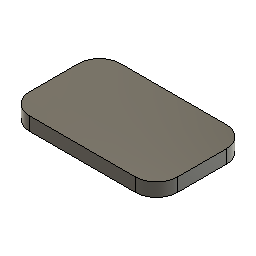
TinyNES_Foam_Cutout_A (Autodesk Fusion 360 design; units mm, degrees)
Autodesk Fusion 360 part; units mm, degrees
sketch "Sketch1" plane through (0, 0, 0) normal (0, 1, 0) x (1, 0, 0)
  line L0 (0, 0) -> (170, 0)
  line L1 (170, 0) -> (170, 170)
  line L2 (170, 170) -> (0, 170)
  line L3 (0, 170) -> (0, 0)
  line L4 (85, 170) -> (85, 128.5) construction
  line L5 (110, 107) -> (60, 107)
  line L6 (50, 117) -> (50, 140)
  line L7 (60, 150) -> (110, 150)
  line L8 (120, 140) -> (120, 117)
  line L9 (120, 107) -> (50, 150) construction
  line L10 (50, 107) -> (120, 150) construction
  arc A0 (60, 150) -> (50, 140) centre (60, 140) ccw
  arc A1 (120, 140) -> (110, 150) centre (110, 140) ccw
  arc A2 (110, 107) -> (120, 117) centre (110, 117) ccw
  arc A3 (50, 117) -> (60, 107) centre (60, 117) ccw
  line L11 (85, 128.5) -> (0, 128.5) construction
  line L12 (85, 128.5) -> (170, 128.5) construction
  arc A4 (0, 108.5) -> (0, 148.5) centre (0, 128.5) ccw
  arc A5 (170, 148.5) -> (170, 108.5) centre (170, 128.5) ccw
  line L13 (85, 0) -> (85, 53.5) construction
  line L14 (140, 20) -> (30, 20)
  line L15 (20, 30) -> (20, 87)
  line L16 (20, 87) -> (150, 87)
  line L17 (150, 87) -> (150, 30)
  line L18 (150, 20) -> (20, 87) construction
  line L19 (20, 20) -> (150, 87) construction
  arc A6 (20, 30) -> (30, 20) centre (30, 30) ccw
  arc A7 (140, 20) -> (150, 30) centre (140, 30) ccw
  line L20 (85, 53.5) -> (20, 53.5) construction
  line L21 (85, 53.5) -> (150, 53.5) construction
  line L22 (20, 53.5) -> (13.5, 53.5) construction
  line L23 (13.5, 53.5) -> (13.5, 64)
  line L24 (13.5, 53.5) -> (13.5, 43)
  line L25 (13.5, 43) -> (13.5, 36.5) construction
  line L26 (13.5, 36.5) -> (20, 36.5) construction
  line L27 (13.5, 64) -> (13.5, 70.5) construction
  line L28 (13.5, 70.5) -> (20, 70.5) construction
  line L29 (13.5, 64) -> (20, 70.5)
  line L30 (13.5, 43) -> (20, 36.5)
  line L31 (156.5, 64) -> (150, 70.5)
  line L32 (156.5, 53.5) -> (156.5, 64)
  line L33 (156.5, 53.5) -> (156.5, 43)
  line L34 (156.5, 43) -> (150, 36.5)
  line L35 (20, 87) -> (20, 85) construction
  line L36 (20, 85) -> (30, 85) construction
  arc A8 (37.0711, 92.0711) -> (20, 85) centre (30, 85) ccw
  line L37 (30, 85) -> (37.0711, 92.0711) construction
  line L38 (30, 85) -> (20, 85) construction
  line L39 (37.0711, 92.0711) -> (42.1421, 87)
  arc A9 (150, 85) -> (132.9289, 92.0711) centre (140, 85) ccw
  line L40 (132.9289, 92.0711) -> (127.8579, 87)
  point P0 (85, 128.5)
  point P1 (85, 53.5)
  dimension "d1" = 170
  dimension "d2" = 170
  dimension "d19" = 41.5
  dimension "d20" = 70
  dimension "d21" = 43
  dimension "d22" = 10
  dimension "d23" = 10
  dimension "d24" = 10
  dimension "d25" = 10
  dimension "d26" = 20
  dimension "d27" = 20
  dimension "d28" = 53.5
  dimension "d29" = 130
  dimension "d30" = 67
  dimension "d31" = 10
  dimension "d32" = 10
  dimension "d33" = 6.5
  dimension "d34" = 10.5
  dimension "d35" = 10.5
  dimension "d36" = 6.5
  dimension "d37" = 6.5
  dimension "d38" = 2
  dimension "d39" = 10
  dimension "d40" = 135
  constraint horizontal L0
  constraint vertical L1
  constraint horizontal L2
  constraint vertical L3
  constraint coincident L0.start L3.end
  constraint midpoint L2 L4.start
  constraint perpendicular L2 L4
  constraint horizontal L5
  constraint perpendicular L5 L6
  constraint parallel L5 L7
  constraint parallel L6 L8
  constraint coincident L9 P0
  constraint coincident L10 P0
  constraint coincident P0 L4.end
  constraint coincident L9.end L6
  constraint coincident L9.end L7
  constraint tangent L6 A0
  constraint tangent L7 A0
  constraint coincident L10.end L7
  constraint coincident L10.end L8
  constraint tangent L7 A1
  constraint tangent L8 A1
  constraint coincident L9.start L8
  constraint coincident L9.start L5
  constraint tangent L8 A2
  constraint tangent L5 A2
  constraint coincident L10.start L6
  constraint coincident L10.start L5
  constraint tangent L6 A3
  constraint tangent L5 A3
  constraint coincident L3 L11.end
  constraint perpendicular L3 L11
  constraint coincident L1 L12.end
  constraint perpendicular L1 L12
  constraint coincident L11.end A4.centre
  constraint coincident L12.end A5.centre
  constraint midpoint L0 L13.start
  constraint perpendicular L0 L13
  constraint horizontal L14
  constraint perpendicular L14 L15
  constraint parallel L14 L16
  constraint parallel L15 L17
  constraint coincident L18 P1
  constraint coincident L19 P1
  constraint coincident P1 L13.end
  constraint coincident L19.start L15
  constraint coincident L19.start L14
  constraint tangent L15 A6
  constraint tangent L14 A6
  constraint coincident L18.start L14
  constraint coincident L18.start L17
  constraint tangent L14 A7
  constraint tangent L17 A7
  constraint coincident L15 L20.end
  constraint perpendicular L15 L20
  constraint coincident L17 L21.end
  constraint perpendicular L17 L21
  constraint perpendicular L15 L22
  constraint perpendicular L22 L23
  constraint perpendicular L22 L24
  constraint parallel L24 L25
  constraint coincident L15 L26.end
  constraint perpendicular L15 L26
  constraint perpendicular L22 L27
  constraint coincident L15 L28.end
  constraint perpendicular L15 L28
  constraint symmetric L13 L22.end L32.start
  constraint symmetric L13 L23.end L31.start
  constraint symmetric L13 L24.end L33.end
  constraint symmetric L13 L26.end L34.end
  constraint symmetric L13 L28.end L31.end
  constraint perpendicular L16 L35
  constraint perpendicular L15 L36
  constraint coincident L36.end A8.centre
  constraint coincident L16 L39.end
  constraint tangent A8 L39
  constraint symmetric L13 L35.end A9.start
  constraint symmetric L13 A8.start A9.end
  constraint symmetric L13 A8 A9
  constraint symmetric L13 L39.end L40.end
  measures "d1" distance of L0.start L0.end
  measures "d2" distance of L0.start L2.end
  measures "d19" distance of L4.start P0
  measures "d20" distance of L9.end L10.end
  measures "d21" distance of L10.start L9.end
  measures "d22" radius of A0
  measures "d23" radius of A1
  measures "d24" radius of A2
  measures "d25" radius of A3
  measures "d26" radius of A4
  measures "d27" radius of A5
  measures "d28" distance of L13.start P1
  measures "d29" distance of L15.end L16.end
  measures "d30" distance of L19.start L15.end
  measures "d31" radius of A6
  measures "d32" radius of A7
  measures "d33" distance of L20.end L22.end
  measures "d34" distance of L22.end L23.end
  measures "d35" distance of L22.end L24.end
  measures "d36" distance of L24.end L25.end
  measures "d37" distance of L23.end L27.end
  measures "d38" distance of L15.end L35.end
  measures "d39" distance of L35.end L36.end
  measures "d40" angle of L37 L38
extrude "Extrude1" add sketch "Sketch1" along normal blind 6.35 contours L5 L6 L7 L8 A0 A1 A2 A3
